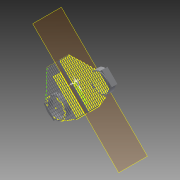
# Autodesk Inventor part: LauncherBase
Saved by Autodesk Inventor 2014 SP1 (Build 180222100, 222)
## iProperties
Created: 2015-03-25
Part Number: LauncherBase
Material: Generic
Document SubType Name: Modeling
Designer: Eric
Density: 1 g/cm^3
Appearance: Default
Author: Eric
Autodesk Inventor part; units mm, degrees
(part 1 of 2)
ref_plane "YZ Plane" through (0, 0, 0) normal (1, 0, 0) x (0, 1, 0)
ref_plane "XZ Plane" through (0, 0, 0) normal (0, 1, 0) x (-1, 0, 0)
ref_plane "XY Plane" through (0, 0, 0) normal (0, 0, 1) x (1, 0, 0)
sketch "Sketch1" plane through (0, 0, 0) normal (0, 1, 0) x (-1, 0, 0)
  line L0 (-54.5, -54.5) -> (54.5, -54.5)
  line L1 (54.5, -54.5) -> (54.5, 54.5)
  line L2 (54.5, 54.5) -> (-54.5, 54.5)
  line L3 (-54.5, 54.5) -> (-54.5, -54.5)
  line L4 (-54.5, -54.5) -> (54.5, 54.5) construction
  line L5 (54.5, -54.5) -> (-54.5, 54.5) construction
  point P0 (0, 0)
  dimension "d0" = 109
  dimension "d1" = 109
  constraints: 12 end point, 2 midpoint, 2 parallel, 1 horizontal, 1 perpendicular
  measures "d0" distance of L2.end L1.end
  measures "d1" distance of L0.end L1.end
extrude "Extrusion1" add sketch "Sketch1" against normal blind 1
sketch "Sketch2" plane through (0, 0, 0) normal (0, 1, 0) x (1, 0, 0)
  circle A0 centre (-31.4663, 31.4663) radius 12.5
  circle A1 centre (0, 0) radius 20 construction
  circle A2 centre (-31.4663, 31.4663) radius 25 construction
  line L0 (-54.5, 54.5) -> (54.5, -54.5) construction
  arc A3 (-45.4655, 31.3234) -> (-31.3234, 45.4655) centre (-31.4663, 31.4663) ccw
  line L1 (-54.5, -54.5) -> (54.5, 54.5) construction
  circle A4 centre (31.4663, -31.4663) radius 12.5
  line L2 (-41.3657, 41.3657) -> (-34.2947, 48.4368)
  line L3 (-34.2947, 48.4368) -> (-31.3234, 45.4655)
  line L4 (-41.3657, 41.3657) -> (-48.4368, 34.2947)
  line L5 (-48.4368, 34.2947) -> (-45.4655, 31.3234)
  line L6 (41.3657, -41.3657) -> (48.4368, -34.2947)
  line L7 (48.4368, -34.2947) -> (45.4655, -31.3234)
  line L8 (41.3657, -41.3657) -> (34.2947, -48.4368)
  line L9 (34.2947, -48.4368) -> (31.3234, -45.4655)
  arc A5 (45.4655, -31.3234) -> (31.3234, -45.4655) centre (31.4663, -31.4663) ccw
  dimension "d4" = 25
  dimension "d6" = 40
  dimension "d7" = 50
  dimension "d8" = 44.5
  dimension "d9" = 1.5
  dimension "d47" = 10
  constraints: 20 end point, 9 symmetric about line, 6 centre point, 4 point on circle, 3 coincident, 2 perpendicular, 2 point on line, 1 tangent, 1 other
  measures "d4" diameter of A0
  measures "d6" diameter of A1
  measures "d7" diameter of A2
  measures "d8" distance of point (0, 0) A0.centre
  measures "d9" radial gap between concentric circles of A0 A3
  measures "d47" distance between parallel lines of L0 L3
extrude "Extrusion2" add sketch "Sketch2" along normal blind 8
sketch "Sketch3" plane through (0, 0, 0) normal (0, 1, 0) x (1, 0, 0)
  circle A0 centre (-31.4663, 31.4663) radius 14 projected
  circle A1 centre (0, 0) radius 20 construction
  circle A2 centre (-31.4663, 31.4663) radius 25 construction
  line L0 (-54.5, -54.5) -> (54.5, 54.5) construction
  line L1 (54.5, -54.5) -> (-54.5, 54.5) construction
  line L2 (-43.1335, -13.435) -> (-0.7071, 28.9914)
  line L3 (-28.2843, -28.2843) -> (-37.6304, -18.9382) construction
  circle A3 centre (31.4663, -31.4663) radius 14 projected
  line L4 (-43.1335, -13.435) -> (-43.8406, -12.7279)
  line L5 (-43.8406, -12.7279) -> (-1.4142, 29.6985)
  line L6 (-1.4142, 29.6985) -> (-0.7071, 28.9914)
  line L7 (-13.435, -43.1335) -> (28.9914, -0.7071)
  line L8 (-13.435, -43.1335) -> (-12.7279, -43.8406)
  line L9 (-12.7279, -43.8406) -> (29.6985, -1.4142)
  line L10 (29.6985, -1.4142) -> (28.9914, -0.7071)
  dimension "d12" = 40
  dimension "d13" = 50
  dimension "d14" = 21
  dimension "d16" = 0
  dimension "d17" = 40
  dimension "d18" = 60
  dimension "d19" = 1
  constraints: 22 end point, 5 symmetric about line, 3 parallel, 3 perpendicular, 3 point on line, 2 centre point, 2 coincident, 1 collinear
  measures "d12" diameter of A1
  measures "d13" diameter of A2
  measures "d14" distance between parallel lines of L0 L2
  measures "d16" angle of L3 L1
  measures "d17" distance from line of point (0, 0) L3
  measures "d18" distance of L2.start L2.end
  measures "d19" distance of L5.end L6.end
extrude "Extrusion3" [suppressed]
sketch "Sketch5" plane through (-43.8406, 0, 12.7279) normal (-0.7071068, 0, -0.7071068) x (-0.7071068, 0, 0.7071068)
  line L0 (0, 0) -> (-60, 0) projected
  line L1 (0, 0) -> (0, 31) projected
  line L2 (-60, 0) -> (-60, 31) projected
  line L3 (-55.2569, 8) -> (-20.5399, 8) construction
  line L4 (-52.3968, 7) -> (-24.3968, 7)
  line L5 (-55.2569, 30) -> (-20.5399, 30) construction
  line L6 (-52.3968, 7) -> (-52.3968, 27)
  line L7 (-52.3968, 27) -> (-52.3968, 7)
  arc A0 (-38.3968, 30) -> (-52.3968, 27) centre (-38.3968, -4.1667) ccw
  line L8 (-38.3968, 7) -> (-38.3968, 32.1795) construction
  circle A1 centre (-38.3968, 20) radius 20 construction
  line L9 (-40, 0) -> (37.0746, 0) construction
  line L10 (-52.3968, 7) -> (-52.3968, 0)
  line L11 (-52.3968, 0) -> (-38.3968, 0) construction
  line L12 (-52.3968, 0) -> (-38.3968, 0)
  line L13 (-24.3968, 7) -> (-24.3968, 27)
  arc A2 (-24.3968, 27) -> (-38.3968, 30) centre (-38.3968, -4.1667) ccw
  line L14 (-24.3968, 7) -> (-24.3968, 0)
  line L15 (-24.3968, 0) -> (-38.3968, 0) construction
  line L16 (-38.3968, 0) -> (-24.3968, 0)
  point P0 (-40, 0)
  dimension "d29" = 40
  dimension "d22" = 8
  dimension "d23" = 28
  dimension "d24" = 14
  dimension "d25" = 30
  dimension "d26" = 20
  dimension "d27" = 14
  dimension "d28" = 7.6032
  constraints: 26 end point, 5 point on line, 4 parallel, 4 point on circle, 3 collinear, 3 horizontal, 3 perpendicular, 2 centre point, 2 symmetric about line, 1 midpoint, 1 tangent, 1 vertical alignment, 3 other
  measures "d22" distance between parallel lines of L0 L3
  measures "d23" distance of L4.start L4.end
  measures "d24" distance of L4.start L8.start
  measures "d25" distance between parallel lines of L0 L5
  measures "d26" distance of L4.start L6.end
  measures "d27" diameter of L0 L4
  measures "d28" distance between parallel lines of L6 L2
extrude "Extrusion4" [suppressed]
sketch "Sketch6" plane through (0, 0, 0) normal (0, 1, 0) x (1, 0, 0)
  line L0 (29.6985, -1.4142) -> (-12.7279, -43.8406) projected
  circle A0 centre (-31.4663, 31.4663) radius 14 projected
  line L1 (-43.8406, -12.7279) -> (-45.4567, 30.9486)
  line L2 (-1.4142, 29.6985) -> (-24.2389, 43.4565)
  circle A1 centre (-31.4663, 31.4663) radius 14 projected
  line L3 (-0.7071, 28.9914) -> (28.9914, -0.7071)
  line L4 (-43.1335, -13.435) -> (-13.435, -43.1335)
  line L5 (-54.5, -54.5) -> (54.5, 54.5) construction
  line L6 (-12.7279, -43.8406) -> (30.9486, -45.4567)
  line L7 (29.6985, -1.4142) -> (43.4565, -24.2389)
  point P0 (0, 0)
  constraints: 14 end point, 2 perpendicular, 2 point on circle, 2 symmetric about line, 2 tangent, 1 parallel
ref_plane "Work Plane1" through (-54.5, 0, 54.5) normal (0.7071068, 0, 0.7071068) x (0.7071068, 0, -0.7071068)
mirror "Mirror1" [suppressed]
sketch "Sketch7" plane through (0, 0, 0) normal (0, 1, 0) x (1, 0, 0)
  line L0 (23.6151, -6.0833) -> (28.9914, -0.7071) projected
  line L1 (28.9914, -0.7071) -> (29.6985, -1.4142) projected
  line L2 (29.6985, -1.4142) -> (24.3222, -6.7905) projected
  line L3 (24.3222, -6.7905) -> (23.6151, -6.0833) projected
  line L4 (4.5233, -26.5894) -> (3.8161, -25.8823) projected
  line L5 (4.5233, -26.5894) -> (-12.7279, -43.8406) projected
  line L6 (-12.7279, -43.8406) -> (-13.435, -43.1335) projected
  line L7 (-13.435, -43.1335) -> (3.8161, -25.8823) projected
  line L8 (-6.7905, 24.3222) -> (-1.4142, 29.6985) projected
  line L9 (-1.4142, 29.6985) -> (-0.7071, 28.9914) projected
  line L10 (-0.7071, 28.9914) -> (-6.0833, 23.6151) projected
  line L11 (-6.7905, 24.3222) -> (-6.0833, 23.6151) projected
  line L12 (-26.5894, 4.5233) -> (-25.8823, 3.8161) projected
  line L13 (-25.8823, 3.8161) -> (-43.1335, -13.435) projected
  line L14 (-43.1335, -13.435) -> (-43.8406, -12.7279) projected
  line L15 (-43.8406, -12.7279) -> (-26.5894, 4.5233) projected
  circle A0 centre (-31.4663, 31.4663) radius 14 projected
  circle A1 centre (31.4663, -31.4663) radius 14 projected
  line L16 (54.5, 54.5) -> (-54.5, 54.5) projected
  line L17 (-54.5, 54.5) -> (-54.5, -54.5) projected
  line L18 (-54.5, -54.5) -> (54.5, -54.5) projected
  line L19 (54.5, -54.5) -> (54.5, 54.5) projected
  line L20 (-1.4142, 29.6985) -> (-24.2389, 43.4565)
  line L21 (-0.7071, 28.9914) -> (28.9914, -0.7071)
  line L22 (29.6985, -1.4142) -> (43.4565, -24.2389)
  line L23 (-12.7279, -43.8406) -> (30.9486, -45.4567)
  line L24 (-13.435, -43.1335) -> (-43.1335, -13.435)
  line L25 (-43.8406, -12.7279) -> (-45.4567, 30.9486)
  point P0 (0, 0)
  constraints: 12 end point, 4 point on circle, 4 tangent, 1 parallel, 1 perpendicular
extrude "Extrusion5" cut sketch "Sketch7" against normal blind 2
sketch "Sketch8" plane through (-43.1335, 0, 13.435) normal (-0.7071068, 0, 0.7071068) x (0.7071068, 0, 0.7071068)
  line L0 (0, 0) -> (0, 31) projected
  line L1 (-1, 31) -> (0, 31) projected
  line L2 (-1, 0) -> (-1, 31) projected
  line L3 (-1, 0) -> (-1, -2) projected
  line L4 (43, -2) -> (-1, -2) projected
  line L5 (43, 0) -> (43, -2) projected
  line L6 (43, 0) -> (43, 31) projected
  line L7 (42, 31) -> (43, 31) projected
  line L8 (42, 0) -> (42, 31) projected
  line L9 (0, 0) -> (42, 0) projected
  circle A0 centre (21, 20) radius 20
  point P0 (21, 0)
  dimension "d35" = 40
  constraints: 1 centre point, 1 tangent
  measures "d35" diameter of A0
sketch "Sketch9" plane through (-6.7905, 0, -24.3222) normal (-0.7071068, 0, -0.7071068) x (-0.7071068, 0, 0.7071068)
  line L0 (52.3968, 0) -> (28, 0) projected
  line L1 (52.3968, 0) -> (52.3968, 31) projected
  line L2 (0, 0) -> (-7.6032, 0) projected
  line L3 (29.4896, 11.5) -> (47.4982, 11.5) construction
  arc A0 (39.8968, 11.5) -> (31, 0) centre (45.8259, -2.2785) ccw
  arc A1 (49.3968, 0) -> (39.8968, 11.5) centre (34.6132, -2.5386) ccw
  line L4 (28, 0) -> (52.3968, 0) projected
  line L5 (31, 0) -> (49.3968, 0) construction
  point P0 (12.3968, 0)
  dimension "d36" = 3
  dimension "d37" = 3
  dimension "d38" = 11.5
  dimension "d39" = 12.5
  dimension "d40" = 15
  constraints: 4 end point, 4 point on circle, 3 point on line, 2 centre point, 1 collinear, 1 equal radius, 1 parallel
  measures "d36" distance of L0.start L5.end
  measures "d37" distance of L5.start L0.end
  measures "d38" distance between parallel lines of L4 L3
  measures "d39" distance from line of L1 A0.start
  measures "d40" radius of A1
extrude "Extrusion6" [suppressed]
mirror "Mirror2" [suppressed]
sketch "Sketch10" plane through (0, 0, 0) normal (0, 1, 0) x (1, 0, 0)
  arc A0 (-45.4567, 30.9486) -> (-24.2389, 43.4565) centre (-31.4663, 31.4663) ccw projected
  line L0 (-30.3601, 17.51) -> (-33.8925, 18.5492)
  line L1 (-39.9536, 20.3323) -> (-39.4963, 21.8867)
  line L2 (-39.4963, 21.8867) -> (-29.9028, 19.0644)
  line L3 (-29.9028, 19.0644) -> (-30.3601, 17.51)
  line L4 (-40.5117, 19.5635) -> (-30.5117, 16.5635) construction
  line L5 (-30.5117, 19.5635) -> (-40.5117, 16.5635) construction
  circle A1 centre (-31.4663, 31.4663) radius 12.5 projected
  circle A2 centre (-31.4663, 31.4663) radius 14 projected
  arc A3 (-39.9536, 20.3323) -> (-30.3601, 17.51) centre (-31.4663, 31.4663) ccw
  point P0 (0, 0)
  point P1 (-35.5117, 18.0635)
  dimension "d43" = 10
  constraints: 12 end point, 6 point on circle, 2 midpoint, 2 parallel, 1 centre point, 1 perpendicular, 1 point on line
  measures "d43" distance of L1.end L2.end
extrude "Extrusion7" cut sketch "Sketch10" along normal blind 2 contours L1 A1 L3 A0
mirror "Mirror3" about plane through (-54.5, 0, 54.5) normal (0.7071068, 0, 0.7071068) of "Extrusion7"
sketch "Sketch13" plane through (0, 0, 0) normal (0, 1, 0) x (1, 0, 0)
  line L0 (-43.8406, -12.7279) -> (-12.7279, -43.8406) projected
  line L1 (29.6985, -1.4142) -> (-1.4142, 29.6985) projected
  line L2 (14.1421, 14.1421) -> (-28.2843, -28.2843) construction
  line L3 (-30.052, -26.5165) -> (12.3744, 15.9099)
  line L4 (12.3744, 15.9099) -> (15.9099, 12.3744)
  line L5 (15.9099, 12.3744) -> (-26.5165, -30.052)
  line L6 (-26.5165, -30.052) -> (-30.052, -26.5165)
  point P0 (0, 0)
  point P1 (-7.0711, -7.0711)
  dimension "d49" = 5
  dimension "d50" = 2.5
  constraints: 10 end point, 3 midpoint, 2 collinear, 2 parallel, 2 perpendicular
  measures "d49" distance of L3.end L4.end
  measures "d50" distance between parallel lines of L5 L2
extrude "Extrusion8" cut sketch "Sketch13" against normal blind 0.25
sketch "Sketch15" plane through (0, 0, 0) normal (0, 1, 0) x (1, 0, 0)
  line L0 (-30.052, -26.5165) -> (12.3744, 15.9099) projected
  line L1 (12.3744, 15.9099) -> (-1.4142, 29.6985) projected
  line L2 (-43.8406, -12.7279) -> (-30.052, -26.5165) projected
  line L3 (10.9602, 15.9099) -> (8.8388, 13.7886)
  line L4 (8.8388, 13.7886) -> (6.7175, 15.9099)
  line L5 (6.7175, 15.9099) -> (8.8388, 18.0312)
  line L6 (8.8388, 18.0312) -> (10.9602, 15.9099)
  point P0 (0, 0)
  dimension "d72" = 3
  dimension "d73" = 3
  dimension "d74" = 1
  dimension "d75" = 1
  constraints: 8 end point, 5 parallel
  measures "d72" distance of L4.end L5.end
  measures "d73" distance of L3.end L4.end
  measures "d74" distance between parallel lines of L1 L6
  measures "d75" distance between parallel lines of L0 L3
extrude "Extrusion9" cut sketch "Sketch15" against normal blind 5
pattern_linear "Rectangular Pattern1" count 17 spacing 3.45 along (-0.7071068, 0, 0.7071068) count 15 spacing 3.45 along (-0.7071068, 0, -0.7071068) of "Extrusion9"
mirror "Mirror4" about plane through (-54.5, 0, 54.5) normal (0.7071068, 0, 0.7071068) of "Extrusion9", "Rectangular Pattern1"
sketch "Sketch16" plane through (0, 0, 0) normal (0, 1, 0) x (1, 0, 0)
  line L0 (-5.4801, 23.2285) -> (-3.3588, 25.3498) projected
  line L1 (-30.052, -26.5165) -> (12.3744, 15.9099) projected
  line L2 (12.3744, 15.9099) -> (-1.4142, 29.6985) projected
  line L3 (-3.0406, 27.0822) -> (-4.4548, 25.668)
  line L4 (-4.4548, 25.668) -> (-6.3866, 26.1856)
  line L5 (-6.3866, 26.1856) -> (-6.9043, 28.1175)
  line L6 (-6.9043, 28.1175) -> (-5.49, 29.5317)
  line L7 (-5.49, 29.5317) -> (-3.5582, 29.014)
  line L8 (-3.5582, 29.014) -> (-3.0406, 27.0822)
  line L9 (-4.9724, 27.5998) -> (-6.1972, 28.8246) construction
  line L10 (-4.9724, 27.5998) -> (-6.6454, 27.1515) construction
  point P0 (0, 0)
  dimension "d84" = 1
  dimension "d85" = 4
  dimension "d87" = 2
  constraints: 16 end point, 2 midpoint, 1 parallel, 13 other
  measures "d84" distance between parallel lines of L0 L3
  measures "d85" distance from line of L2 L9.start
  measures "d87" distance of L3.end L4.end
extrude "Extrusion10" [suppressed]
sketch "Sketch17" plane through (0, 0, 0) normal (0, 1, 0) x (1, 0, 0)
  line L0 (-32.633, -3.9244) -> (-30.5117, -6.0458) projected
  line L1 (-30.5117, -6.0458) -> (-32.633, -8.1671) projected
  line L2 (-32.633, -8.1671) -> (-34.7543, -6.0458) projected
  line L3 (-34.7543, -6.0458) -> (-32.633, -3.9244) projected
  line L4 (-30.1935, -1.4849) -> (-28.0721, -3.6062) projected
  line L5 (-28.0721, -3.6062) -> (-30.1935, -5.7276) projected
  line L6 (-30.1935, -5.7276) -> (-32.3148, -3.6062) projected
  line L7 (-32.3148, -3.6062) -> (-30.1935, -1.4849) projected
  line L8 (-27.7539, 0.9546) -> (-25.6326, -1.1667) projected
  line L9 (-25.6326, -1.1667) -> (-27.7539, -3.288) projected
  line L10 (-27.7539, -3.288) -> (-29.8753, -1.1667) projected
  line L11 (-29.8753, -1.1667) -> (-27.7539, 0.9546) projected
  line L12 (-25.3144, 3.3941) -> (-23.1931, 1.2728) projected
  line L13 (-23.1931, 1.2728) -> (-25.3144, -0.8485) projected
  line L14 (-25.3144, -0.8485) -> (-27.4357, 1.2728) projected
  line L15 (-27.4357, 1.2728) -> (-25.3144, 3.3941) projected
  line L16 (-22.8749, 5.8336) -> (-20.7536, 3.7123) projected
  line L17 (-20.7536, 3.7123) -> (-22.8749, 1.591) projected
  line L18 (-22.8749, 1.591) -> (-24.9962, 3.7123) projected
  line L19 (-24.9962, 3.7123) -> (-22.8749, 5.8336) projected
  line L20 (-20.4354, 8.2731) -> (-18.3141, 6.1518) projected
  line L21 (-18.3141, 6.1518) -> (-20.4354, 4.0305) projected
  line L22 (-20.4354, 4.0305) -> (-22.5567, 6.1518) projected
  line L23 (-22.5567, 6.1518) -> (-20.4354, 8.2731) projected
  line L24 (-17.9959, 10.7127) -> (-15.8745, 8.5913) projected
  line L25 (-15.8745, 8.5913) -> (-17.9959, 6.47) projected
  line L26 (-17.9959, 6.47) -> (-20.1172, 8.5913) projected
  line L27 (-20.1172, 8.5913) -> (-17.9959, 10.7127) projected
  line L28 (-15.5563, 13.1522) -> (-13.435, 11.0309) projected
  line L29 (-13.435, 11.0309) -> (-15.5563, 8.9095) projected
  line L30 (-15.5563, 8.9095) -> (-17.6777, 11.0309) projected
  line L31 (-17.6777, 11.0309) -> (-15.5563, 13.1522) projected
  line L32 (-13.1168, 15.5917) -> (-10.9955, 13.4704) projected
  line L33 (-10.9955, 13.4704) -> (-13.1168, 11.3491) projected
  line L34 (-13.1168, 11.3491) -> (-15.2382, 13.4704) projected
  line L35 (-15.2382, 13.4704) -> (-13.1168, 15.5917) projected
  line L36 (-10.6773, 18.0312) -> (-8.556, 15.9099) projected
  line L37 (-8.556, 15.9099) -> (-10.6773, 13.7886) projected
  line L38 (-10.6773, 13.7886) -> (-12.7986, 15.9099) projected
  line L39 (-12.7986, 15.9099) -> (-10.6773, 18.0312) projected
  line L40 (-8.2378, 20.4707) -> (-6.1165, 18.3494) projected
  line L41 (-6.1165, 18.3494) -> (-8.2378, 16.2281) projected
  line L42 (-8.2378, 16.2281) -> (-10.3591, 18.3494) projected
  line L43 (-10.3591, 18.3494) -> (-8.2378, 20.4707) projected
  line L44 (-5.7983, 22.9103) -> (-3.677, 20.7889) projected
  line L45 (-3.677, 20.7889) -> (-5.7983, 18.6676) projected
  line L46 (-5.7983, 18.6676) -> (-7.9196, 20.7889) projected
  line L47 (-7.9196, 20.7889) -> (-5.7983, 22.9103) projected
  line L48 (-3.3588, 25.3498) -> (-1.2374, 23.2285) projected
  line L49 (-1.2374, 23.2285) -> (-3.3588, 21.1071) projected
  line L50 (-3.3588, 21.1071) -> (-5.4801, 23.2285) projected
  line L51 (-5.4801, 23.2285) -> (-3.3588, 25.3498) projected
  line L52 (-0.9192, 27.7893) -> (1.2021, 25.668) projected
  line L53 (1.2021, 25.668) -> (-0.9192, 23.5467) projected
  line L54 (-0.9192, 23.5467) -> (-3.0406, 25.668) projected
  line L55 (-3.0406, 25.668) -> (-0.9192, 27.7893) projected
  line L56 (-30.1935, -6.364) -> (-28.0721, -8.4853) projected
  line L57 (-28.0721, -8.4853) -> (-30.1935, -10.6066) projected
  line L58 (-30.1935, -10.6066) -> (-32.3148, -8.4853) projected
  line L59 (-32.3148, -8.4853) -> (-30.1935, -6.364) projected
  line L60 (-27.7539, -3.9244) -> (-25.6326, -6.0458) projected
  line L61 (-25.6326, -6.0458) -> (-27.7539, -8.1671) projected
  line L62 (-27.7539, -8.1671) -> (-29.8753, -6.0458) projected
  line L63 (-29.8753, -6.0458) -> (-27.7539, -3.9244) projected
  line L64 (-25.3144, -1.4849) -> (-23.1931, -3.6062) projected
  line L65 (-23.1931, -3.6062) -> (-25.3144, -5.7276) projected
  line L66 (-25.3144, -5.7276) -> (-27.4357, -3.6062) projected
  line L67 (-27.4357, -3.6062) -> (-25.3144, -1.4849) projected
  line L68 (-22.8749, 0.9546) -> (-20.7536, -1.1667) projected
  line L69 (-20.7536, -1.1667) -> (-22.8749, -3.288) projected
  line L70 (-22.8749, -3.288) -> (-24.9962, -1.1667) projected
  line L71 (-24.9962, -1.1667) -> (-22.8749, 0.9546) projected
  line L72 (-20.4354, 3.3941) -> (-18.3141, 1.2728) projected
  line L73 (-18.3141, 1.2728) -> (-20.4354, -0.8485) projected
  line L74 (-20.4354, -0.8485) -> (-22.5567, 1.2728) projected
  line L75 (-22.5567, 1.2728) -> (-20.4354, 3.3941) projected
  line L76 (-17.9959, 5.8336) -> (-15.8745, 3.7123) projected
  line L77 (-15.8745, 3.7123) -> (-17.9959, 1.591) projected
  line L78 (-17.9959, 1.591) -> (-20.1172, 3.7123) projected
  line L79 (-20.1172, 3.7123) -> (-17.9959, 5.8336) projected
  line L80 (-15.5563, 8.2731) -> (-13.435, 6.1518) projected
  line L81 (-13.435, 6.1518) -> (-15.5563, 4.0305) projected
  line L82 (-15.5563, 4.0305) -> (-17.6777, 6.1518) projected
  line L83 (-17.6777, 6.1518) -> (-15.5563, 8.2731) projected
  line L84 (-13.1168, 10.7127) -> (-10.9955, 8.5913) projected
  line L85 (-10.9955, 8.5913) -> (-13.1168, 6.47) projected
  line L86 (-13.1168, 6.47) -> (-15.2382, 8.5913) projected
  line L87 (-15.2382, 8.5913) -> (-13.1168, 10.7127) projected
  line L88 (-10.6773, 13.1522) -> (-8.556, 11.0309) projected
  line L89 (-8.556, 11.0309) -> (-10.6773, 8.9095) projected
  line L90 (-10.6773, 8.9095) -> (-12.7986, 11.0309) projected
  line L91 (-12.7986, 11.0309) -> (-10.6773, 13.1522) projected
  line L92 (-8.2378, 15.5917) -> (-6.1165, 13.4704) projected
  line L93 (-6.1165, 13.4704) -> (-8.2378, 11.3491) projected
  line L94 (-8.2378, 11.3491) -> (-10.3591, 13.4704) projected
  line L95 (-10.3591, 13.4704) -> (-8.2378, 15.5917) projected
  line L96 (-5.7983, 18.0312) -> (-3.677, 15.9099) projected
  line L97 (-3.677, 15.9099) -> (-5.7983, 13.7886) projected
  line L98 (-5.7983, 13.7886) -> (-7.9196, 15.9099) projected
  line L99 (-7.9196, 15.9099) -> (-5.7983, 18.0312) projected
  line L100 (-3.3588, 20.4707) -> (-1.2374, 18.3494) projected
  line L101 (-1.2374, 18.3494) -> (-3.3588, 16.2281) projected
  line L102 (-3.3588, 16.2281) -> (-5.4801, 18.3494) projected
  line L103 (-5.4801, 18.3494) -> (-3.3588, 20.4707) projected
  line L104 (-0.9192, 22.9103) -> (1.2021, 20.7889) projected
  line L105 (1.2021, 20.7889) -> (-0.9192, 18.6676) projected
  line L106 (-0.9192, 18.6676) -> (-3.0406, 20.7889) projected
  line L107 (-3.0406, 20.7889) -> (-0.9192, 22.9103) projected
  line L108 (1.5203, 25.3498) -> (3.6416, 23.2285) projected
  line L109 (3.6416, 23.2285) -> (1.5203, 21.1071) projected
  line L110 (1.5203, 21.1071) -> (-0.601, 23.2285) projected
  line L111 (-0.601, 23.2285) -> (1.5203, 25.3498) projected
  line L112 (-27.7539, -8.8035) -> (-25.6326, -10.9248) projected
  line L113 (-25.6326, -10.9248) -> (-27.7539, -13.0461) projected
  line L114 (-27.7539, -13.0461) -> (-29.8753, -10.9248) projected
  line L115 (-29.8753, -10.9248) -> (-27.7539, -8.8035) projected
  line L116 (-25.3144, -6.364) -> (-23.1931, -8.4853) projected
  line L117 (-23.1931, -8.4853) -> (-25.3144, -10.6066) projected
  line L118 (-25.3144, -10.6066) -> (-27.4357, -8.4853) projected
  line L119 (-27.4357, -8.4853) -> (-25.3144, -6.364) projected
  line L120 (-22.8749, -3.9244) -> (-20.7536, -6.0458) projected
  line L121 (-20.7536, -6.0458) -> (-22.8749, -8.1671) projected
  line L122 (-22.8749, -8.1671) -> (-24.9962, -6.0458) projected
  line L123 (-24.9962, -6.0458) -> (-22.8749, -3.9244) projected
  line L124 (-20.4354, -1.4849) -> (-18.3141, -3.6062) projected
  line L125 (-18.3141, -3.6062) -> (-20.4354, -5.7276) projected
  line L126 (-20.4354, -5.7276) -> (-22.5567, -3.6062) projected
  line L127 (-22.5567, -3.6062) -> (-20.4354, -1.4849) projected
  line L128 (-17.9959, 0.9546) -> (-15.8745, -1.1667) projected
  line L129 (-15.8745, -1.1667) -> (-17.9959, -3.288) projected
  line L130 (-17.9959, -3.288) -> (-20.1172, -1.1667) projected
  line L131 (-20.1172, -1.1667) -> (-17.9959, 0.9546) projected
  line L132 (-15.5563, 3.3941) -> (-13.435, 1.2728) projected
  line L133 (-13.435, 1.2728) -> (-15.5563, -0.8485) projected
  line L134 (-15.5563, -0.8485) -> (-17.6777, 1.2728) projected
  line L135 (-17.6777, 1.2728) -> (-15.5563, 3.3941) projected
  line L136 (-13.1168, 5.8336) -> (-10.9955, 3.7123) projected
  line L137 (-10.9955, 3.7123) -> (-13.1168, 1.591) projected
  line L138 (-13.1168, 1.591) -> (-15.2382, 3.7123) projected
  line L139 (-15.2382, 3.7123) -> (-13.1168, 5.8336) projected
  line L140 (-10.6773, 8.2731) -> (-8.556, 6.1518) projected
  line L141 (-8.556, 6.1518) -> (-10.6773, 4.0305) projected
  line L142 (-10.6773, 4.0305) -> (-12.7986, 6.1518) projected
  line L143 (-12.7986, 6.1518) -> (-10.6773, 8.2731) projected
  line L144 (-8.2378, 10.7127) -> (-6.1165, 8.5913) projected
  line L145 (-6.1165, 8.5913) -> (-8.2378, 6.47) projected
  line L146 (-8.2378, 6.47) -> (-10.3591, 8.5913) projected
  line L147 (-10.3591, 8.5913) -> (-8.2378, 10.7127) projected
  line L148 (-5.7983, 13.1522) -> (-3.677, 11.0309) projected
  line L149 (-3.677, 11.0309) -> (-5.7983, 8.9095) projected
  line L150 (-5.7983, 8.9095) -> (-7.9196, 11.0309) projected
  line L151 (-7.9196, 11.0309) -> (-5.7983, 13.1522) projected
  line L152 (-3.3588, 15.5917) -> (-1.2374, 13.4704) projected
  line L153 (-1.2374, 13.4704) -> (-3.3588, 11.3491) projected
  line L154 (-3.3588, 11.3491) -> (-5.4801, 13.4704) projected
  line L155 (-5.4801, 13.4704) -> (-3.3588, 15.5917) projected
  line L156 (-0.9192, 18.0312) -> (1.2021, 15.9099) projected
  line L157 (1.2021, 15.9099) -> (-0.9192, 13.7886) projected
  line L158 (-0.9192, 13.7886) -> (-3.0406, 15.9099) projected
  line L159 (-3.0406, 15.9099) -> (-0.9192, 18.0312) projected
  line L160 (1.5203, 20.4707) -> (3.6416, 18.3494) projected
  line L161 (3.6416, 18.3494) -> (1.5203, 16.2281) projected
  line L162 (1.5203, 16.2281) -> (-0.601, 18.3494) projected
  line L163 (-0.601, 18.3494) -> (1.5203, 20.4707) projected
  line L164 (3.9598, 22.9103) -> (6.0811, 20.7889) projected
  line L165 (6.0811, 20.7889) -> (3.9598, 18.6676) projected
  line L166 (3.9598, 18.6676) -> (1.8385, 20.7889) projected
  line L167 (1.8385, 20.7889) -> (3.9598, 22.9103) projected
  line L168 (-25.3144, -11.243) -> (-23.1931, -13.3643) projected
  line L169 (-23.1931, -13.3643) -> (-25.3144, -15.4856) projected
  line L170 (-25.3144, -15.4856) -> (-27.4357, -13.3643) projected
  line L171 (-27.4357, -13.3643) -> (-25.3144, -11.243) projected
  line L172 (-22.8749, -8.8035) -> (-20.7536, -10.9248) projected
  line L173 (-20.7536, -10.9248) -> (-22.8749, -13.0461) projected
  line L174 (-22.8749, -13.0461) -> (-24.9962, -10.9248) projected
  line L175 (-24.9962, -10.9248) -> (-22.8749, -8.8035) projected
  line L176 (-20.4354, -6.364) -> (-18.3141, -8.4853) projected
  line L177 (-18.3141, -8.4853) -> (-20.4354, -10.6066) projected
  line L178 (-20.4354, -10.6066) -> (-22.5567, -8.4853) projected
  line L179 (-22.5567, -8.4853) -> (-20.4354, -6.364) projected
  line L180 (-17.9959, -3.9244) -> (-15.8745, -6.0458) projected
  line L181 (-15.8745, -6.0458) -> (-17.9959, -8.1671) projected
  line L182 (-17.9959, -8.1671) -> (-20.1172, -6.0458) projected
  line L183 (-20.1172, -6.0458) -> (-17.9959, -3.9244) projected
  line L184 (-15.5563, -1.4849) -> (-13.435, -3.6062) projected
  line L185 (-13.435, -3.6062) -> (-15.5563, -5.7276) projected
  line L186 (-15.5563, -5.7276) -> (-17.6777, -3.6062) projected
  line L187 (-17.6777, -3.6062) -> (-15.5563, -1.4849) projected
  line L188 (-13.1168, 0.9546) -> (-10.9955, -1.1667) projected
  line L189 (-10.9955, -1.1667) -> (-13.1168, -3.288) projected
  line L190 (-13.1168, -3.288) -> (-15.2382, -1.1667) projected
  line L191 (-15.2382, -1.1667) -> (-13.1168, 0.9546) projected
  line L192 (-10.6773, 3.3941) -> (-8.556, 1.2728) projected
  line L193 (-8.556, 1.2728) -> (-10.6773, -0.8485) projected
  line L194 (-10.6773, -0.8485) -> (-12.7986, 1.2728) projected
  line L195 (-12.7986, 1.2728) -> (-10.6773, 3.3941) projected
  line L196 (-8.2378, 5.8336) -> (-6.1165, 3.7123) projected
  line L197 (-6.1165, 3.7123) -> (-8.2378, 1.591) projected
  line L198 (-8.2378, 1.591) -> (-10.3591, 3.7123) projected
  line L199 (-10.3591, 3.7123) -> (-8.2378, 5.8336) projected
  line L200 (-5.7983, 8.2731) -> (-3.677, 6.1518) projected
  line L201 (-3.677, 6.1518) -> (-5.7983, 4.0305) projected
  line L202 (-5.7983, 4.0305) -> (-7.9196, 6.1518) projected
  line L203 (-7.9196, 6.1518) -> (-5.7983, 8.2731) projected
  line L204 (-3.3588, 10.7127) -> (-1.2374, 8.5913) projected
  line L205 (-1.2374, 8.5913) -> (-3.3588, 6.47) projected
  line L206 (-3.3588, 6.47) -> (-5.4801, 8.5913) projected
  line L207 (-5.4801, 8.5913) -> (-3.3588, 10.7127) projected
  line L208 (-0.9192, 13.1522) -> (1.2021, 11.0309) projected
  line L209 (1.2021, 11.0309) -> (-0.9192, 8.9095) projected
  line L210 (-0.9192, 8.9095) -> (-3.0406, 11.0309) projected
  line L211 (-3.0406, 11.0309) -> (-0.9192, 13.1522) projected
  line L212 (1.5203, 15.5917) -> (3.6416, 13.4704) projected
  line L213 (3.6416, 13.4704) -> (1.5203, 11.3491) projected
  line L214 (1.5203, 11.3491) -> (-0.601, 13.4704) projected
  line L215 (-0.601, 13.4704) -> (1.5203, 15.5917) projected
  line L216 (3.9598, 18.0312) -> (6.0811, 15.9099) projected
  line L217 (6.0811, 15.9099) -> (3.9598, 13.7886) projected
  line L218 (3.9598, 13.7886) -> (1.8385, 15.9099) projected
  line L219 (1.8385, 15.9099) -> (3.9598, 18.0312) projected
  line L220 (6.3993, 20.4707) -> (8.5206, 18.3494) projected
  line L221 (8.5206, 18.3494) -> (6.3993, 16.2281) projected
  line L222 (6.3993, 16.2281) -> (4.278, 18.3494) projected
  line L223 (4.278, 18.3494) -> (6.3993, 20.4707) projected
  line L224 (-22.8749, -13.6825) -> (-20.7536, -15.8038) projected
  line L225 (-20.7536, -15.8038) -> (-22.8749, -17.9252) projected
  line L226 (-22.8749, -17.9252) -> (-24.9962, -15.8038) projected
  line L227 (-24.9962, -15.8038) -> (-22.8749, -13.6825) projected
  line L228 (-20.4354, -11.243) -> (-18.3141, -13.3643) projected
  line L229 (-18.3141, -13.3643) -> (-20.4354, -15.4856) projected
  line L230 (-20.4354, -15.4856) -> (-22.5567, -13.3643) projected
  line L231 (-22.5567, -13.3643) -> (-20.4354, -11.243) projected
  line L232 (-17.9959, -8.8035) -> (-15.8745, -10.9248) projected
  line L233 (-15.8745, -10.9248) -> (-17.9959, -13.0461) projected
  line L234 (-17.9959, -13.0461) -> (-20.1172, -10.9248) projected
  line L235 (-20.1172, -10.9248) -> (-17.9959, -8.8035) projected
  line L236 (-15.5563, -6.364) -> (-13.435, -8.4853) projected
  line L237 (-13.435, -8.4853) -> (-15.5563, -10.6066) projected
  line L238 (-15.5563, -10.6066) -> (-17.6777, -8.4853) projected
  line L239 (-17.6777, -8.4853) -> (-15.5563, -6.364) projected
  line L240 (-13.1168, -3.9244) -> (-10.9955, -6.0458) projected
  line L241 (-10.9955, -6.0458) -> (-13.1168, -8.1671) projected
  line L242 (-13.1168, -8.1671) -> (-15.2382, -6.0458) projected
  line L243 (-15.2382, -6.0458) -> (-13.1168, -3.9244) projected
  line L244 (-10.6773, -1.4849) -> (-8.556, -3.6062) projected
  line L245 (-8.556, -3.6062) -> (-10.6773, -5.7276) projected
  line L246 (-10.6773, -5.7276) -> (-12.7986, -3.6062) projected
  line L247 (-12.7986, -3.6062) -> (-10.6773, -1.4849) projected
  line L248 (-8.2378, 0.9546) -> (-6.1165, -1.1667) projected
  line L249 (-6.1165, -1.1667) -> (-8.2378, -3.288) projected
  line L250 (-8.2378, -3.288) -> (-10.3591, -1.1667) projected
  line L251 (-10.3591, -1.1667) -> (-8.2378, 0.9546) projected
  line L252 (-5.7983, 3.3941) -> (-3.677, 1.2728) projected
  line L253 (-3.677, 1.2728) -> (-5.7983, -0.8485) projected
  line L254 (-5.7983, -0.8485) -> (-7.9196, 1.2728) projected
  line L255 (-7.9196, 1.2728) -> (-5.7983, 3.3941) projected
  line L256 (-3.3588, 5.8336) -> (-1.2374, 3.7123) projected
  line L257 (-1.2374, 3.7123) -> (-3.3588, 1.591) projected
  line L258 (-3.3588, 1.591) -> (-5.4801, 3.7123) projected
  line L259 (-5.4801, 3.7123) -> (-3.3588, 5.8336) projected
  line L260 (-0.9192, 8.2731) -> (1.2021, 6.1518) projected
  line L261 (1.2021, 6.1518) -> (-0.9192, 4.0305) projected
  line L262 (-0.9192, 4.0305) -> (-3.0406, 6.1518) projected
  line L263 (-3.0406, 6.1518) -> (-0.9192, 8.2731) projected
  line L264 (1.5203, 10.7127) -> (3.6416, 8.5913) projected
  line L265 (3.6416, 8.5913) -> (1.5203, 6.47) projected
  line L266 (1.5203, 6.47) -> (-0.601, 8.5913) projected
  line L267 (-0.601, 8.5913) -> (1.5203, 10.7127) projected
  line L268 (3.9598, 13.1522) -> (6.0811, 11.0309) projected
  line L269 (6.0811, 11.0309) -> (3.9598, 8.9095) projected
  line L270 (3.9598, 8.9095) -> (1.8385, 11.0309) projected
  line L271 (1.8385, 11.0309) -> (3.9598, 13.1522) projected
  line L272 (6.3993, 15.5917) -> (8.5206, 13.4704) projected
  line L273 (8.5206, 13.4704) -> (6.3993, 11.3491) projected
  line L274 (6.3993, 11.3491) -> (4.278, 13.4704) projected
  line L275 (4.278, 13.4704) -> (6.3993, 15.5917) projected
  line L276 (8.8388, 18.0312) -> (10.9602, 15.9099) projected
  line L277 (10.9602, 15.9099) -> (8.8388, 13.7886) projected
  line L278 (8.8388, 13.7886) -> (6.7175, 15.9099) projected
  line L279 (6.7175, 15.9099) -> (8.8388, 18.0312) projected
  line L280 (-30.052, -26.5165) -> (12.3744, 15.9099) projected
  line L281 (12.3744, 15.9099) -> (-1.4142, 29.6985) projected
  line L282 (-1.4142, 29.6985) -> (-24.2389, 43.4565) projected
  arc A0 (-30.3601, 17.51) -> (-24.2389, 43.4565) centre (-31.4663, 31.4663) ccw projected
  line L283 (-30.3601, 17.51) -> (-29.9028, 19.0644) projected
  arc A1 (-29.9028, 19.0644) -> (-39.4963, 21.8867) centre (-31.4663, 31.4663) ccw projected
  line L284 (-39.4963, 21.8867) -> (-39.9536, 20.3323) projected
  arc A2 (-45.4567, 30.9486) -> (-39.9536, 20.3323) centre (-31.4663, 31.4663) ccw projected
  line L285 (-45.4567, 30.9486) -> (-43.8406, -12.7279) projected
  line L286 (-43.8406, -12.7279) -> (-30.052, -26.5165) projected
  point P0 (0, 0)
sketch "Sketch18" plane through (0, 0, 0) normal (0, 1, 0) x (1, 0, 0)
  line L0 (15.9099, 10.9602) -> (18.0312, 8.8388) projected
  line L1 (18.0312, 8.8388) -> (15.9099, 6.7175) projected
  line L2 (15.9099, 6.7175) -> (13.7886, 8.8388) projected
  line L3 (13.7886, 8.8388) -> (15.9099, 10.9602) projected
  line L4 (13.4704, 8.5206) -> (15.5917, 6.3993) projected
  line L5 (15.5917, 6.3993) -> (13.4704, 4.278) projected
  line L6 (13.4704, 4.278) -> (11.3491, 6.3993) projected
  line L7 (11.3491, 6.3993) -> (13.4704, 8.5206) projected
  line L8 (11.0309, 6.0811) -> (13.1522, 3.9598) projected
  line L9 (13.1522, 3.9598) -> (11.0309, 1.8385) projected
  line L10 (11.0309, 1.8385) -> (8.9095, 3.9598) projected
  line L11 (8.9095, 3.9598) -> (11.0309, 6.0811) projected
  line L12 (8.5913, 3.6416) -> (10.7127, 1.5203) projected
  line L13 (10.7127, 1.5203) -> (8.5913, -0.601) projected
  line L14 (8.5913, -0.601) -> (6.47, 1.5203) projected
  line L15 (6.47, 1.5203) -> (8.5913, 3.6416) projected
  line L16 (6.1518, 1.2021) -> (8.2731, -0.9192) projected
  line L17 (8.2731, -0.9192) -> (6.1518, -3.0406) projected
  line L18 (6.1518, -3.0406) -> (4.0305, -0.9192) projected
  line L19 (4.0305, -0.9192) -> (6.1518, 1.2021) projected
  line L20 (3.7123, -1.2374) -> (5.8336, -3.3588) projected
  line L21 (5.8336, -3.3588) -> (3.7123, -5.4801) projected
  line L22 (3.7123, -5.4801) -> (1.591, -3.3588) projected
  line L23 (1.591, -3.3588) -> (3.7123, -1.2374) projected
  line L24 (1.2728, -3.677) -> (3.3941, -5.7983) projected
  line L25 (3.3941, -5.7983) -> (1.2728, -7.9196) projected
  line L26 (1.2728, -7.9196) -> (-0.8485, -5.7983) projected
  line L27 (-0.8485, -5.7983) -> (1.2728, -3.677) projected
  line L28 (-1.1667, -6.1165) -> (0.9546, -8.2378) projected
  line L29 (0.9546, -8.2378) -> (-1.1667, -10.3591) projected
  line L30 (-1.1667, -10.3591) -> (-3.288, -8.2378) projected
  line L31 (-3.288, -8.2378) -> (-1.1667, -6.1165) projected
  line L32 (-3.6062, -8.556) -> (-1.4849, -10.6773) projected
  line L33 (-1.4849, -10.6773) -> (-3.6062, -12.7986) projected
  line L34 (-3.6062, -12.7986) -> (-5.7276, -10.6773) projected
  line L35 (-5.7276, -10.6773) -> (-3.6062, -8.556) projected
  line L36 (-6.0458, -10.9955) -> (-3.9244, -13.1168) projected
  line L37 (-3.9244, -13.1168) -> (-6.0458, -15.2382) projected
  line L38 (-6.0458, -15.2382) -> (-8.1671, -13.1168) projected
  line L39 (-8.1671, -13.1168) -> (-6.0458, -10.9955) projected
  line L40 (-8.4853, -13.435) -> (-6.364, -15.5563) projected
  line L41 (-6.364, -15.5563) -> (-8.4853, -17.6777) projected
  line L42 (-8.4853, -17.6777) -> (-10.6066, -15.5563) projected
  line L43 (-10.6066, -15.5563) -> (-8.4853, -13.435) projected
  line L44 (-10.9248, -15.8745) -> (-8.8035, -17.9959) projected
  line L45 (-8.8035, -17.9959) -> (-10.9248, -20.1172) projected
  line L46 (-10.9248, -20.1172) -> (-13.0461, -17.9959) projected
  line L47 (-13.0461, -17.9959) -> (-10.9248, -15.8745) projected
  line L48 (-13.3643, -18.3141) -> (-11.243, -20.4354) projected
  line L49 (-11.243, -20.4354) -> (-13.3643, -22.5567) projected
  line L50 (-13.3643, -22.5567) -> (-15.4856, -20.4354) projected
  line L51 (-15.4856, -20.4354) -> (-13.3643, -18.3141) projected
  line L52 (-15.8038, -20.7536) -> (-13.6825, -22.8749) projected
  line L53 (-13.6825, -22.8749) -> (-15.8038, -24.9962) projected
  line L54 (-15.8038, -24.9962) -> (-17.9252, -22.8749) projected
  line L55 (-17.9252, -22.8749) -> (-15.8038, -20.7536) projected
  line L56 (-18.2434, -23.1931) -> (-16.122, -25.3144) projected
  line L57 (-16.122, -25.3144) -> (-18.2434, -27.4357) projected
  line L58 (-18.2434, -27.4357) -> (-20.3647, -25.3144) projected
  line L59 (-20.3647, -25.3144) -> (-18.2434, -23.1931) projected
  line L60 (-20.6829, -25.6326) -> (-18.5616, -27.7539) projected
  line L61 (-18.5616, -27.7539) -> (-20.6829, -29.8753) projected
  line L62 (-20.6829, -29.8753) -> (-22.8042, -27.7539) projected
  line L63 (-22.8042, -27.7539) -> (-20.6829, -25.6326) projected
  line L64 (-23.1224, -28.0721) -> (-21.0011, -30.1935) projected
  line L65 (-21.0011, -30.1935) -> (-23.1224, -32.3148) projected
  line L66 (-23.1224, -32.3148) -> (-25.2437, -30.1935) projected
  line L67 (-25.2437, -30.1935) -> (-23.1224, -28.0721) projected
  line L68 (18.3494, 8.5206) -> (20.4707, 6.3993) projected
  line L69 (20.4707, 6.3993) -> (18.3494, 4.278) projected
  line L70 (18.3494, 4.278) -> (16.2281, 6.3993) projected
  line L71 (16.2281, 6.3993) -> (18.3494, 8.5206) projected
  line L72 (15.9099, 6.0811) -> (18.0312, 3.9598) projected
  line L73 (18.0312, 3.9598) -> (15.9099, 1.8385) projected
  line L74 (15.9099, 1.8385) -> (13.7886, 3.9598) projected
  line L75 (13.7886, 3.9598) -> (15.9099, 6.0811) projected
  line L76 (13.4704, 3.6416) -> (15.5917, 1.5203) projected
  line L77 (15.5917, 1.5203) -> (13.4704, -0.601) projected
  line L78 (13.4704, -0.601) -> (11.3491, 1.5203) projected
  line L79 (11.3491, 1.5203) -> (13.4704, 3.6416) projected
  line L80 (11.0309, 1.2021) -> (13.1522, -0.9192) projected
  line L81 (13.1522, -0.9192) -> (11.0309, -3.0406) projected
  line L82 (11.0309, -3.0406) -> (8.9095, -0.9192) projected
  line L83 (8.9095, -0.9192) -> (11.0309, 1.2021) projected
  line L84 (8.5913, -1.2374) -> (10.7127, -3.3588) projected
  line L85 (10.7127, -3.3588) -> (8.5913, -5.4801) projected
  line L86 (8.5913, -5.4801) -> (6.47, -3.3588) projected
  line L87 (6.47, -3.3588) -> (8.5913, -1.2374) projected
  line L88 (6.1518, -3.677) -> (8.2731, -5.7983) projected
  line L89 (8.2731, -5.7983) -> (6.1518, -7.9196) projected
  line L90 (6.1518, -7.9196) -> (4.0305, -5.7983) projected
  line L91 (4.0305, -5.7983) -> (6.1518, -3.677) projected
  line L92 (3.7123, -6.1165) -> (5.8336, -8.2378) projected
  line L93 (5.8336, -8.2378) -> (3.7123, -10.3591) projected
  line L94 (3.7123, -10.3591) -> (1.591, -8.2378) projected
  line L95 (1.591, -8.2378) -> (3.7123, -6.1165) projected
  line L96 (1.2728, -8.556) -> (3.3941, -10.6773) projected
  line L97 (3.3941, -10.6773) -> (1.2728, -12.7986) projected
  line L98 (1.2728, -12.7986) -> (-0.8485, -10.6773) projected
  line L99 (-0.8485, -10.6773) -> (1.2728, -8.556) projected
  line L100 (-1.1667, -10.9955) -> (0.9546, -13.1168) projected
  line L101 (0.9546, -13.1168) -> (-1.1667, -15.2382) projected
  line L102 (-1.1667, -15.2382) -> (-3.288, -13.1168) projected
  line L103 (-3.288, -13.1168) -> (-1.1667, -10.9955) projected
  line L104 (-3.6062, -13.435) -> (-1.4849, -15.5563) projected
  line L105 (-1.4849, -15.5563) -> (-3.6062, -17.6777) projected
  line L106 (-3.6062, -17.6777) -> (-5.7276, -15.5563) projected
  line L107 (-5.7276, -15.5563) -> (-3.6062, -13.435) projected
  line L108 (-6.0458, -15.8745) -> (-3.9244, -17.9959) projected
  line L109 (-3.9244, -17.9959) -> (-6.0458, -20.1172) projected
  line L110 (-6.0458, -20.1172) -> (-8.1671, -17.9959) projected
  line L111 (-8.1671, -17.9959) -> (-6.0458, -15.8745) projected
  line L112 (-8.4853, -18.3141) -> (-6.364, -20.4354) projected
  line L113 (-6.364, -20.4354) -> (-8.4853, -22.5567) projected
  line L114 (-8.4853, -22.5567) -> (-10.6066, -20.4354) projected
  line L115 (-10.6066, -20.4354) -> (-8.4853, -18.3141) projected
  line L116 (-10.9248, -20.7536) -> (-8.8035, -22.8749) projected
  line L117 (-8.8035, -22.8749) -> (-10.9248, -24.9962) projected
  line L118 (-10.9248, -24.9962) -> (-13.0461, -22.8749) projected
  line L119 (-13.0461, -22.8749) -> (-10.9248, -20.7536) projected
  line L120 (-13.3643, -23.1931) -> (-11.243, -25.3144) projected
  line L121 (-11.243, -25.3144) -> (-13.3643, -27.4357) projected
  line L122 (-13.3643, -27.4357) -> (-15.4856, -25.3144) projected
  line L123 (-15.4856, -25.3144) -> (-13.3643, -23.1931) projected
  line L124 (-15.8038, -25.6326) -> (-13.6825, -27.7539) projected
  line L125 (-13.6825, -27.7539) -> (-15.8038, -29.8753) projected
  line L126 (-15.8038, -29.8753) -> (-17.9252, -27.7539) projected
  line L127 (-17.9252, -27.7539) -> (-15.8038, -25.6326) projected
  line L128 (-18.2434, -28.0721) -> (-16.122, -30.1935) projected
  line L129 (-16.122, -30.1935) -> (-18.2434, -32.3148) projected
  line L130 (-18.2434, -32.3148) -> (-20.3647, -30.1935) projected
  line L131 (-20.3647, -30.1935) -> (-18.2434, -28.0721) projected
  line L132 (-20.6829, -30.5117) -> (-18.5616, -32.633) projected
  line L133 (-18.5616, -32.633) -> (-20.6829, -34.7543) projected
  line L134 (-20.6829, -34.7543) -> (-22.8042, -32.633) projected
  line L135 (-22.8042, -32.633) -> (-20.6829, -30.5117) projected
  line L136 (20.7889, 6.0811) -> (22.9103, 3.9598) projected
  line L137 (22.9103, 3.9598) -> (20.7889, 1.8385) projected
  line L138 (20.7889, 1.8385) -> (18.6676, 3.9598) projected
  line L139 (18.6676, 3.9598) -> (20.7889, 6.0811) projected
  line L140 (18.3494, 3.6416) -> (20.4707, 1.5203) projected
  line L141 (20.4707, 1.5203) -> (18.3494, -0.601) projected
  line L142 (18.3494, -0.601) -> (16.2281, 1.5203) projected
  line L143 (16.2281, 1.5203) -> (18.3494, 3.6416) projected
  line L144 (15.9099, 1.2021) -> (18.0312, -0.9192) projected
  line L145 (18.0312, -0.9192) -> (15.9099, -3.0406) projected
  line L146 (15.9099, -3.0406) -> (13.7886, -0.9192) projected
  line L147 (13.7886, -0.9192) -> (15.9099, 1.2021) projected
  line L148 (13.4704, -1.2374) -> (15.5917, -3.3588) projected
  line L149 (15.5917, -3.3588) -> (13.4704, -5.4801) projected
  line L150 (13.4704, -5.4801) -> (11.3491, -3.3588) projected
  line L151 (11.3491, -3.3588) -> (13.4704, -1.2374) projected
  line L152 (11.0309, -3.677) -> (13.1522, -5.7983) projected
  line L153 (13.1522, -5.7983) -> (11.0309, -7.9196) projected
  line L154 (11.0309, -7.9196) -> (8.9095, -5.7983) projected
  line L155 (8.9095, -5.7983) -> (11.0309, -3.677) projected
  line L156 (8.5913, -6.1165) -> (10.7127, -8.2378) projected
  line L157 (10.7127, -8.2378) -> (8.5913, -10.3591) projected
  line L158 (8.5913, -10.3591) -> (6.47, -8.2378) projected
  line L159 (6.47, -8.2378) -> (8.5913, -6.1165) projected
  line L160 (6.1518, -8.556) -> (8.2731, -10.6773) projected
  line L161 (8.2731, -10.6773) -> (6.1518, -12.7986) projected
  line L162 (6.1518, -12.7986) -> (4.0305, -10.6773) projected
  line L163 (4.0305, -10.6773) -> (6.1518, -8.556) projected
  line L164 (3.7123, -10.9955) -> (5.8336, -13.1168) projected
  line L165 (5.8336, -13.1168) -> (3.7123, -15.2382) projected
  line L166 (3.7123, -15.2382) -> (1.591, -13.1168) projected
  line L167 (1.591, -13.1168) -> (3.7123, -10.9955) projected
  line L168 (1.2728, -13.435) -> (3.3941, -15.5563) projected
  line L169 (3.3941, -15.5563) -> (1.2728, -17.6777) projected
  line L170 (1.2728, -17.6777) -> (-0.8485, -15.5563) projected
  line L171 (-0.8485, -15.5563) -> (1.2728, -13.435) projected
  line L172 (-1.1667, -15.8745) -> (0.9546, -17.9959) projected
  line L173 (0.9546, -17.9959) -> (-1.1667, -20.1172) projected
  line L174 (-1.1667, -20.1172) -> (-3.288, -17.9959) projected
  line L175 (-3.288, -17.9959) -> (-1.1667, -15.8745) projected
  line L176 (-3.6062, -18.3141) -> (-1.4849, -20.4354) projected
  line L177 (-1.4849, -20.4354) -> (-3.6062, -22.5567) projected
  line L178 (-3.6062, -22.5567) -> (-5.7276, -20.4354) projected
  line L179 (-5.7276, -20.4354) -> (-3.6062, -18.3141) projected
  line L180 (-6.0458, -20.7536) -> (-3.9244, -22.8749) projected
  line L181 (-3.9244, -22.8749) -> (-6.0458, -24.9962) projected
  line L182 (-6.0458, -24.9962) -> (-8.1671, -22.8749) projected
  line L183 (-8.1671, -22.8749) -> (-6.0458, -20.7536) projected
  line L184 (-8.4853, -23.1931) -> (-6.364, -25.3144) projected
  line L185 (-6.364, -25.3144) -> (-8.4853, -27.4357) projected
  line L186 (-8.4853, -27.4357) -> (-10.6066, -25.3144) projected
  line L187 (-10.6066, -25.3144) -> (-8.4853, -23.1931) projected
  line L188 (-10.9248, -25.6326) -> (-8.8035, -27.7539) projected
  line L189 (-8.8035, -27.7539) -> (-10.9248, -29.8753) projected
  line L190 (-10.9248, -29.8753) -> (-13.0461, -27.7539) projected
  line L191 (-13.0461, -27.7539) -> (-10.9248, -25.6326) projected
  line L192 (-13.3643, -28.0721) -> (-11.243, -30.1935) projected
  line L193 (-11.243, -30.1935) -> (-13.3643, -32.3148) projected
  line L194 (-13.3643, -32.3148) -> (-15.4856, -30.1935) projected
  line L195 (-15.4856, -30.1935) -> (-13.3643, -28.0721) projected
  line L196 (-15.8038, -30.5117) -> (-13.6825, -32.633) projected
  line L197 (-13.6825, -32.633) -> (-15.8038, -34.7543) projected
  line L198 (-15.8038, -34.7543) -> (-17.9252, -32.633) projected
  line L199 (-17.9252, -32.633) -> (-15.8038, -30.5117) projected
  line L200 (-18.2434, -32.9512) -> (-16.122, -35.0725) projected
  line L201 (-16.122, -35.0725) -> (-18.2434, -37.1938) projected
  line L202 (-18.2434, -37.1938) -> (-20.3647, -35.0725) projected
  line L203 (-20.3647, -35.0725) -> (-18.2434, -32.9512) projected
  line L204 (23.2285, 3.6416) -> (25.3498, 1.5203) projected
  line L205 (25.3498, 1.5203) -> (23.2285, -0.601) projected
  line L206 (23.2285, -0.601) -> (21.1071, 1.5203) projected
  line L207 (21.1071, 1.5203) -> (23.2285, 3.6416) projected
  line L208 (20.7889, 1.2021) -> (22.9103, -0.9192) projected
  line L209 (22.9103, -0.9192) -> (20.7889, -3.0406) projected
  line L210 (20.7889, -3.0406) -> (18.6676, -0.9192) projected
  line L211 (18.6676, -0.9192) -> (20.7889, 1.2021) projected
  line L212 (18.3494, -1.2374) -> (20.4707, -3.3588) projected
  line L213 (20.4707, -3.3588) -> (18.3494, -5.4801) projected
  line L214 (18.3494, -5.4801) -> (16.2281, -3.3588) projected
  line L215 (16.2281, -3.3588) -> (18.3494, -1.2374) projected
  line L216 (15.9099, -3.677) -> (18.0312, -5.7983) projected
  line L217 (18.0312, -5.7983) -> (15.9099, -7.9196) projected
  line L218 (15.9099, -7.9196) -> (13.7886, -5.7983) projected
  line L219 (13.7886, -5.7983) -> (15.9099, -3.677) projected
  line L220 (13.4704, -6.1165) -> (15.5917, -8.2378) projected
  line L221 (15.5917, -8.2378) -> (13.4704, -10.3591) projected
  line L222 (13.4704, -10.3591) -> (11.3491, -8.2378) projected
  line L223 (11.3491, -8.2378) -> (13.4704, -6.1165) projected
  line L224 (11.0309, -8.556) -> (13.1522, -10.6773) projected
  line L225 (13.1522, -10.6773) -> (11.0309, -12.7986) projected
  line L226 (11.0309, -12.7986) -> (8.9095, -10.6773) projected
  line L227 (8.9095, -10.6773) -> (11.0309, -8.556) projected
  line L228 (8.5913, -10.9955) -> (10.7127, -13.1168) projected
  line L229 (10.7127, -13.1168) -> (8.5913, -15.2382) projected
  line L230 (8.5913, -15.2382) -> (6.47, -13.1168) projected
  line L231 (6.47, -13.1168) -> (8.5913, -10.9955) projected
  line L232 (6.1518, -13.435) -> (8.2731, -15.5563) projected
  line L233 (8.2731, -15.5563) -> (6.1518, -17.6777) projected
  line L234 (6.1518, -17.6777) -> (4.0305, -15.5563) projected
  line L235 (4.0305, -15.5563) -> (6.1518, -13.435) projected
  line L236 (3.7123, -15.8745) -> (5.8336, -17.9959) projected
  line L237 (5.8336, -17.9959) -> (3.7123, -20.1172) projected
  line L238 (3.7123, -20.1172) -> (1.591, -17.9959) projected
  line L239 (1.591, -17.9959) -> (3.7123, -15.8745) projected
  line L240 (1.2728, -18.3141) -> (3.3941, -20.4354) projected
  line L241 (3.3941, -20.4354) -> (1.2728, -22.5567) projected
  line L242 (1.2728, -22.5567) -> (-0.8485, -20.4354) projected
  line L243 (-0.8485, -20.4354) -> (1.2728, -18.3141) projected
  line L244 (-1.1667, -20.7536) -> (0.9546, -22.8749) projected
  line L245 (0.9546, -22.8749) -> (-1.1667, -24.9962) projected
  line L246 (-1.1667, -24.9962) -> (-3.288, -22.8749) projected
  line L247 (-3.288, -22.8749) -> (-1.1667, -20.7536) projected
  line L248 (-3.6062, -23.1931) -> (-1.4849, -25.3144) projected
  line L249 (-1.4849, -25.3144) -> (-3.6062, -27.4357) projected
  line L250 (-3.6062, -27.4357) -> (-5.7276, -25.3144) projected
  line L251 (-5.7276, -25.3144) -> (-3.6062, -23.1931) projected
  line L252 (-6.0458, -25.6326) -> (-3.9244, -27.7539) projected
  line L253 (-3.9244, -27.7539) -> (-6.0458, -29.8753) projected
  line L254 (-6.0458, -29.8753) -> (-8.1671, -27.7539) projected
  line L255 (-8.1671, -27.7539) -> (-6.0458, -25.6326) projected
  line L256 (-8.4853, -28.0721) -> (-6.364, -30.1935) projected
  line L257 (-6.364, -30.1935) -> (-8.4853, -32.3148) projected
  line L258 (-8.4853, -32.3148) -> (-10.6066, -30.1935) projected
  line L259 (-10.6066, -30.1935) -> (-8.4853, -28.0721) projected
  line L260 (-10.9248, -30.5117) -> (-8.8035, -32.633) projected
  line L261 (-8.8035, -32.633) -> (-10.9248, -34.7543) projected
  line L262 (-10.9248, -34.7543) -> (-13.0461, -32.633) projected
  line L263 (-13.0461, -32.633) -> (-10.9248, -30.5117) projected
  line L264 (-13.3643, -32.9512) -> (-11.243, -35.0725) projected
  line L265 (-11.243, -35.0725) -> (-13.3643, -37.1938) projected
  line L266 (-13.3643, -37.1938) -> (-15.4856, -35.0725) projected
  line L267 (-15.4856, -35.0725) -> (-13.3643, -32.9512) projected
  line L268 (-15.8038, -35.3907) -> (-13.6825, -37.512) projected
  line L269 (-13.6825, -37.512) -> (-15.8038, -39.6333) projected
  line L270 (-15.8038, -39.6333) -> (-17.9252, -37.512) projected
  line L271 (-17.9252, -37.512) -> (-15.8038, -35.3907) projected
  line L272 (25.668, 1.2021) -> (27.7893, -0.9192) projected
  line L273 (27.7893, -0.9192) -> (25.668, -3.0406) projected
  line L274 (25.668, -3.0406) -> (23.5467, -0.9192) projected
  line L275 (23.5467, -0.9192) -> (25.668, 1.2021) projected
  line L276 (23.2285, -1.2374) -> (25.3498, -3.3588) projected
  line L277 (25.3498, -3.3588) -> (23.2285, -5.4801) projected
  line L278 (23.2285, -5.4801) -> (21.1071, -3.3588) projected
  line L279 (21.1071, -3.3588) -> (23.2285, -1.2374) projected
  line L280 (20.7889, -3.677) -> (22.9103, -5.7983) projected
  line L281 (22.9103, -5.7983) -> (20.7889, -7.9196) projected
  line L282 (20.7889, -7.9196) -> (18.6676, -5.7983) projected
  line L283 (18.6676, -5.7983) -> (20.7889, -3.677) projected
  line L284 (18.3494, -6.1165) -> (20.4707, -8.2378) projected
  line L285 (20.4707, -8.2378) -> (18.3494, -10.3591) projected
  line L286 (18.3494, -10.3591) -> (16.2281, -8.2378) projected
  line L287 (16.2281, -8.2378) -> (18.3494, -6.1165) projected
  line L288 (15.9099, -8.556) -> (18.0312, -10.6773) projected
  line L289 (18.0312, -10.6773) -> (15.9099, -12.7986) projected
  line L290 (15.9099, -12.7986) -> (13.7886, -10.6773) projected
  line L291 (13.7886, -10.6773) -> (15.9099, -8.556) projected
  line L292 (13.4704, -10.9955) -> (15.5917, -13.1168) projected
  line L293 (15.5917, -13.1168) -> (13.4704, -15.2382) projected
  line L294 (13.4704, -15.2382) -> (11.3491, -13.1168) projected
  line L295 (11.3491, -13.1168) -> (13.4704, -10.9955) projected
  line L296 (11.0309, -13.435) -> (13.1522, -15.5563) projected
  line L297 (13.1522, -15.5563) -> (11.0309, -17.6777) projected
  line L298 (11.0309, -17.6777) -> (8.9095, -15.5563) projected
  line L299 (8.9095, -15.5563) -> (11.0309, -13.435) projected
  line L300 (8.5913, -15.8745) -> (10.7127, -17.9959) projected
  line L301 (10.7127, -17.9959) -> (8.5913, -20.1172) projected
  line L302 (8.5913, -20.1172) -> (6.47, -17.9959) projected
  line L303 (6.47, -17.9959) -> (8.5913, -15.8745) projected
  line L304 (6.1518, -18.3141) -> (8.2731, -20.4354) projected
  line L305 (8.2731, -20.4354) -> (6.1518, -22.5567) projected
  line L306 (6.1518, -22.5567) -> (4.0305, -20.4354) projected
  line L307 (4.0305, -20.4354) -> (6.1518, -18.3141) projected
  line L308 (3.7123, -20.7536) -> (5.8336, -22.8749) projected
  line L309 (5.8336, -22.8749) -> (3.7123, -24.9962) projected
  line L310 (3.7123, -24.9962) -> (1.591, -22.8749) projected
  line L311 (1.591, -22.8749) -> (3.7123, -20.7536) projected
  line L312 (1.2728, -23.1931) -> (3.3941, -25.3144) projected
  line L313 (3.3941, -25.3144) -> (1.2728, -27.4357) projected
  line L314 (1.2728, -27.4357) -> (-0.8485, -25.3144) projected
  line L315 (-0.8485, -25.3144) -> (1.2728, -23.1931) projected
  line L316 (-1.1667, -25.6326) -> (0.9546, -27.7539) projected
  line L317 (0.9546, -27.7539) -> (-1.1667, -29.8753) projected
  line L318 (-1.1667, -29.8753) -> (-3.288, -27.7539) projected
  line L319 (-3.288, -27.7539) -> (-1.1667, -25.6326) projected
  line L320 (-3.6062, -28.0721) -> (-1.4849, -30.1935) projected
  line L321 (-1.4849, -30.1935) -> (-3.6062, -32.3148) projected
  line L322 (-3.6062, -32.3148) -> (-5.7276, -30.1935) projected
  line L323 (-5.7276, -30.1935) -> (-3.6062, -28.0721) projected
  line L324 (-6.0458, -30.5117) -> (-3.9244, -32.633) projected
  line L325 (-3.9244, -32.633) -> (-6.0458, -34.7543) projected
  line L326 (-6.0458, -34.7543) -> (-8.1671, -32.633) projected
  line L327 (-8.1671, -32.633) -> (-6.0458, -30.5117) projected
  line L328 (-8.4853, -32.9512) -> (-6.364, -35.0725) projected
  line L329 (-6.364, -35.0725) -> (-8.4853, -37.1938) projected
  line L330 (-8.4853, -37.1938) -> (-10.6066, -35.0725) projected
  line L331 (-10.6066, -35.0725) -> (-8.4853, -32.9512) projected
  line L332 (-10.9248, -35.3907) -> (-8.8035, -37.512) projected
  line L333 (-8.8035, -37.512) -> (-10.9248, -39.6333) projected
  line L334 (-10.9248, -39.6333) -> (-13.0461, -37.512) projected
  line L335 (-13.0461, -37.512) -> (-10.9248, -35.3907) projected
  line L336 (-13.3643, -37.8302) -> (-11.243, -39.9515) projected
  line L337 (-11.243, -39.9515) -> (-13.3643, -42.0729) projected
  line L338 (-13.3643, -42.0729) -> (-15.4856, -39.9515) projected
  line L339 (-15.4856, -39.9515) -> (-13.3643, -37.8302) projected
  line L340 (28.1075, -1.2374) -> (30.2288, -3.3588) projected
  line L341 (30.2288, -3.3588) -> (28.1075, -5.4801) projected
  line L342 (28.1075, -5.4801) -> (25.9862, -3.3588) projected
  line L343 (25.9862, -3.3588) -> (28.1075, -1.2374) projected
  line L344 (25.668, -3.677) -> (27.7893, -5.7983) projected
  line L345 (27.7893, -5.7983) -> (25.668, -7.9196) projected
  line L346 (25.668, -7.9196) -> (23.5467, -5.7983) projected
  line L347 (23.5467, -5.7983) -> (25.668, -3.677) projected
  line L348 (23.2285, -6.1165) -> (25.3498, -8.2378) projected
  line L349 (25.3498, -8.2378) -> (23.2285, -10.3591) projected
  line L350 (23.2285, -10.3591) -> (21.1071, -8.2378) projected
  line L351 (21.1071, -8.2378) -> (23.2285, -6.1165) projected
  line L352 (20.7889, -8.556) -> (22.9103, -10.6773) projected
  line L353 (22.9103, -10.6773) -> (20.7889, -12.7986) projected
  line L354 (20.7889, -12.7986) -> (18.6676, -10.6773) projected
  line L355 (18.6676, -10.6773) -> (20.7889, -8.556) projected
  line L356 (18.3494, -10.9955) -> (20.4707, -13.1168) projected
  line L357 (20.4707, -13.1168) -> (18.3494, -15.2382) projected
  line L358 (18.3494, -15.2382) -> (16.2281, -13.1168) projected
  line L359 (16.2281, -13.1168) -> (18.3494, -10.9955) projected
  line L360 (15.9099, -13.435) -> (18.0312, -15.5563) projected
  line L361 (18.0312, -15.5563) -> (15.9099, -17.6777) projected
  line L362 (15.9099, -17.6777) -> (13.7886, -15.5563) projected
  line L363 (13.7886, -15.5563) -> (15.9099, -13.435) projected
  line L364 (13.4704, -15.8745) -> (15.5917, -17.9959) projected
  line L365 (15.5917, -17.9959) -> (13.4704, -20.1172) projected
  line L366 (13.4704, -20.1172) -> (11.3491, -17.9959) projected
  line L367 (11.3491, -17.9959) -> (13.4704, -15.8745) projected
  line L368 (11.0309, -18.3141) -> (13.1522, -20.4354) projected
  line L369 (13.1522, -20.4354) -> (11.0309, -22.5567) projected
  line L370 (11.0309, -22.5567) -> (8.9095, -20.4354) projected
  line L371 (8.9095, -20.4354) -> (11.0309, -18.3141) projected
  line L372 (8.5913, -20.7536) -> (10.7127, -22.8749) projected
  line L373 (10.7127, -22.8749) -> (8.5913, -24.9962) projected
  line L374 (8.5913, -24.9962) -> (6.47, -22.8749) projected
  line L375 (6.47, -22.8749) -> (8.5913, -20.7536) projected